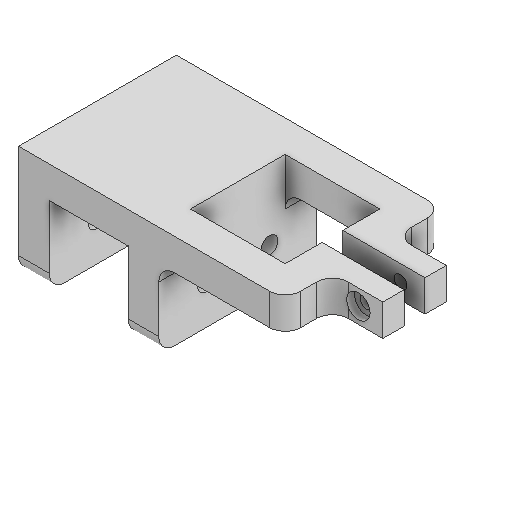
# Autodesk Inventor part: estopMountV1
Saved by Autodesk Inventor 2025 (Build 290162000, 162)
## iProperties
Created: 2024-11-24
Part Number: estopMountV1
Material: Generic
Document SubType Name: Modeling
Designer: derm
Density: 1 g/cm^3
Appearance: Default
Author: derm
Autodesk Inventor part; units mm, degrees
ref_plane "YZ Plane" through (0, 0, 0) normal (1, 0, 0) x (0, 1, 0)
ref_plane "XZ Plane" through (0, 0, 0) normal (0, 1, 0) x (-1, 0, 0)
ref_plane "XY Plane" through (0, 0, 0) normal (0, 0, 1) x (1, 0, 0)
sketch "Sketch1" plane through (0, 0, 0) normal (0, 1, 0) x (-1, 0, 0)
  line L0 (-15, 15) -> (15, 15)
  line L1 (15, 15) -> (15, -15)
  line L2 (15, -15) -> (-15, -15)
  line L3 (-15, 15) -> (15, -15) construction
  line L4 (15, 15) -> (-15, -15) construction
  line L5 (25, 25) -> (-25, 25)
  line L6 (-25, -25) -> (25, -25)
  line L7 (25, 25) -> (59.45, 25)
  line L8 (59.45, 25) -> (59.45, -25)
  line L9 (59.45, -25) -> (25, -25)
  line L10 (-40.9844, -10.0467) -> (-25, -10.0467)
  line L11 (-25, 10.0467) -> (-40.9844, 10.0467)
  line L12 (-40.9844, -10.0467) -> (-20.5822, 10.0467) construction
  line L13 (-27.4388, -3.2939) -> (-40.9844, 10.0467) construction
  line L14 (-40.9844, -3.2939) -> (-15, -3.2939)
  line L15 (-15, 3.2939) -> (-40.9844, 3.2939)
  line L16 (-46.5666, -3.2939) -> (-15, 3.2939) construction
  line L17 (-15, -3.2939) -> (-46.5666, 3.2939) construction
  line L18 (-40.9844, 10.0467) -> (-40.9844, 3.2939)
  line L19 (-40.9844, -3.2939) -> (-40.9844, -10.0467)
  line L20 (-25, 25) -> (-25, 10.0467)
  line L21 (-15, -15) -> (-15, -3.2939)
  line L22 (-15, 3.2939) -> (-15, 15)
  line L23 (-25, -10.0467) -> (-25, -25)
  point P0 (0, 0)
  point P1 (-30.7833, 0)
  dimension "d0" = 30
  dimension "d1" = 30
  dimension "d2" = 10
  dimension "d4" = 44.45
  constraints: 48 end point, 7 parallel, 5 midpoint, 4 horizontal, 2 perpendicular, 2 point on line
  measures "d0" distance of L2.end L0.start
  measures "d1" distance of L1.end L2.end
  measures "d2" distance between parallel lines of L0 L5
  measures "d4" distance between parallel lines of L8 L1
extrude "Extrusion1" add sketch "Sketch1" along normal blind 10
sketch "Sketch2" plane through (0, 0, 0) normal (0, -1, 0) x (1, 0, 0)
  line L0 (15, 15) -> (-15, 15) projected
  line L1 (15, 3.2939) -> (15, 15) projected
  line L2 (40.9844, 3.2939) -> (15, 3.2939) projected
  line L3 (40.9844, 10.0467) -> (40.9844, 3.2939) projected
  line L4 (25, 10.0467) -> (40.9844, 10.0467) projected
  line L5 (25, 25) -> (25, 10.0467) projected
  line L6 (-59.45, 25) -> (25, 25) projected
  line L7 (-59.45, -25) -> (-59.45, 25) projected
  line L8 (25, -25) -> (-59.45, -25) projected
  line L9 (25, -10.0467) -> (25, -25) projected
  line L10 (40.9844, -10.0467) -> (25, -10.0467) projected
  line L11 (40.9844, -3.2939) -> (40.9844, -10.0467) projected
  line L12 (15, -3.2939) -> (40.9844, -3.2939) projected
  line L13 (15, -15) -> (15, -3.2939) projected
  line L14 (-15, -15) -> (15, -15) projected
  line L15 (-15, 15) -> (-15, -15) projected
  line L16 (-49.725, -25) -> (-24.725, -25)
  line L17 (-24.725, -25) -> (-24.725, 25)
  line L18 (-24.725, 25) -> (-49.725, 25)
  line L19 (-49.725, 25) -> (-49.725, -25)
  line L20 (-49.725, -25) -> (-24.725, 25) construction
  line L21 (-24.725, -25) -> (-49.725, 25) construction
  line L22 (-59.45, 25) -> (25, 25) projected
  line L23 (-15, 25) -> (-15, -25)
  line L24 (25, -25) -> (-59.45, -25) projected
  line L25 (-59.45, 25) -> (-49.725, 25)
  line L26 (-59.45, 25) -> (25, 25) projected
  line L27 (-24.725, 25) -> (-15, 25)
  line L28 (-59.45, 21.5922) -> (-49.725, 21.5922)
  line L29 (-24.725, 21.5922) -> (-15, 21.5922)
  line L30 (-15, 15) -> (-15, -15) projected
  point P0 (0, 0)
  point P1 (-37.225, 0)
  point P2 (-15, -25)
  dimension "d7" = 25
  constraints: 22 end point, 9 point on line, 4 collinear, 3 perpendicular, 2 midpoint, 2 parallel, 1 horizontal
  measures "d7" distance between parallel lines of L19 L17
extrude "Extrusion2" add sketch "Sketch2" along normal blind 25 contours L15 L23 L8 L17 L29 | L29 L17 L6 L23 | L8 L7 L28 L19 | L19 L28 L7 L6
sketch "Sketch3" plane through (-24.725, 0, -25) normal (-1, 0, 0) x (0, 0, 1)
  line L0 (0, 0) -> (50, 0) construction
  line L1 (0, 0) -> (0, -25) construction
  line L2 (50, -25) -> (0, -25) construction
  line L3 (50, 0) -> (50, -25) construction
  line L4 (0, -12.5) -> (50, -12.5) construction
  line L5 (50, 0) -> (50, -25) construction
  line L6 (15, -12.5) -> (35, -12.5) construction
  line L7 (15, -15.2) -> (35, -15.2) construction
  line L8 (35, -9.8) -> (15, -9.8) construction
  arc A0 (15, -9.8) -> (15, -15.2) centre (15, -12.5) ccw construction
  arc A1 (35, -15.2) -> (35, -9.8) centre (35, -12.5) ccw
  circle A2 centre (35, -12.5) radius 2.7
  circle A3 centre (15, -12.5) radius 2.7
  point P0 (25, 0)
  point P1 (25, -12.5)
  point P2 (35, -9.8)
  dimension "d10" = 20
  dimension "d11" = 2.7
  constraints: 10 end point, 4 centre point, 4 midpoint, 4 point on circle, 4 tangent, 2 coincident, 1 concentric, 1 parallel, 1 point on line
  measures "d10" distance of L6.start L6.end
  measures "d11" radius of A0
extrude "Extrusion3" cut sketch "Sketch3" along normal through all both and the other way through all
fillet "Fillet1" radius 5 10 edges at (-15, 0, 20) (-15, 0, -20) (25, 5, -25) (25, 5, -10.0467) (25, 5, 10.0467) (25, 5, 25) (-19.8625, -25, 25) (-19.8625, -25, -25) (-54.5875, -25, -25) (-54.5875, -25, 25)
sketch "Sketch4" plane through (40.9844, 0, 10.0467) normal (0, 0, 1) x (1, 0, 0)
  line L0 (-10.9844, 0) -> (-10.9844, 10) projected
  line L1 (-10.9844, 0) -> (0, 0) projected
  line L2 (0, 0) -> (0, 10) projected
  line L3 (-10.9844, 10) -> (0, 10) projected
  circle A0 centre (-7.7256, 5) radius 2
  point P0 (-40.9844, 0)
  dimension "d15" = 4
  constraints: 1 centre point
  measures "d15" diameter of A0
extrude "Extrusion4" cut sketch "Sketch4" against normal through all contours A0
sketch "Sketch5" plane through (40.9844, 0, 10.0467) normal (0, 0, 1) x (1, 0, 0)
  circle A0 centre (-7.7256, 5) radius 2 projected
  circle A1 centre (-7.7256, 5) radius 3.6921
  point P0 (-40.9844, 0)
  constraints: 1 centre point, 1 coincident
extrude "Extrusion5" cut sketch "Sketch5" along normal mid plane 5
body "Solid1"
